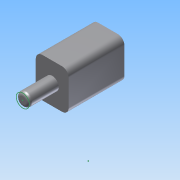
# Autodesk Inventor part: 모터
Saved by Autodesk Inventor 2011 (Build 150239000, 239)
## iProperties
Created: 2019-04-03
Part Number: 모터
Document SubType Name: Modeling
Designer: User
Density: 1 g/cm^3
Author: User
Autodesk Inventor part; units mm, degrees
ref_plane "YZ Plane" through (0, 0, 0) normal (1, 0, 0) x (0, 1, 0)
ref_plane "XZ Plane" through (0, 0, 0) normal (0, 1, 0) x (-1, 0, 0)
ref_plane "XY Plane" through (0, 0, 0) normal (0, 0, 1) x (1, 0, 0)
sketch "스케치1" plane through (0, 0, 0) normal (0, 0, 1) x (1, 0, 0)
  line L0 (-25.0184, 51.8207) -> (-15.0184, 51.8207)
  line L1 (-15.0184, 51.8207) -> (-15.0184, 25.8207)
  line L2 (-15.0184, 25.8207) -> (-25.0184, 25.8207)
  line L3 (-25.0184, 25.8207) -> (-25.0184, 51.8207)
  dimension "d4" = 10
  dimension "d5" = 26
  constraints: 8 end point, 2 parallel, 1 horizontal, 1 perpendicular
  measures "d4" distance of L0.start L0.end
  measures "d5" distance of L2.end L0.start
extrude "돌출1" add sketch "스케치1" along normal blind 12
sketch "스케치2" plane through (-25.0184, 25.8207, 0) normal (0, -1, 0) x (1, 0, 0)
  line L0 (10, 12) -> (0, 12) projected
  line L1 (0, 0) -> (0, 12) projected
  line L2 (10, 0) -> (0, 0) projected
  line L3 (10, 0) -> (10, 12) projected
  line L4 (5, 0) -> (5, 6)
  circle A0 centre (5, 6) radius 2
  point P0 (25.0184, 0)
  dimension "d8" = 4
  constraints: 2 end point, 1 centre point, 1 coincident, 1 midpoint, 1 parallel
  measures "d8" diameter of A0
extrude "돌출2" cut sketch "스케치2" against normal blind 9
sketch "스케치3" plane through (-20.0184, 25.8207, 6) normal (0, -1, 0) x (1, 0, 0)
  circle A0 centre (0, 0) radius 2 projected
  point P0 (20.0184, -6)
fillet "모깎기1" radius 2 4 edges at (-15.0184, 43.3207, 0) (-15.0184, 43.3207, 12) (-25.0184, 43.3207, 12) (-25.0184, 43.3207, 0)
fillet "모깎기2" radius 1 1 edges at (-22.0184, 25.8207, 6)
